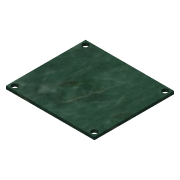
# Autodesk Inventor part: 00_motordriver_pcb
Saved by Autodesk Inventor 2019.4 (Build 234330000, 330)
## iProperties
Created: 2020-06-15
Part Number: 00_motordriver_pcb
Material: Generic
Document SubType Name: Modeling
Designer: diederichbenedict
Density: 1 g/cm^3
Appearance: Green Polished
Author: diederichbenedict
Autodesk Inventor part; units mm, degrees
ref_plane "YZ Plane" through (0, 0, 0) normal (1, 0, 0) x (0, 1, 0)
ref_plane "XZ Plane" through (0, 0, 0) normal (0, 1, 0) x (-1, 0, 0)
ref_plane "XY Plane" through (0, 0, 0) normal (0, 0, 1) x (1, 0, 0)
sketch "Sketch1" plane through (0, 0, 0) normal (0, 1, 0) x (-1, 0, 0)
  line L0 (0, 0) -> (-30, 0)
  line L1 (-30, 0) -> (-30, 27)
  line L2 (-30, 27) -> (0, 27)
  line L3 (0, 27) -> (0, 0)
  dimension "d0" = 30
  dimension "d1" = 27
  constraints: 8 end point, 2 parallel, 1 horizontal, 1 perpendicular
  measures "d0" distance of L1.end L2.end
  measures "d1" distance of L0.end L1.end
extrude "Extrusion1" add sketch "Sketch1" along normal blind 1
sketch "Sketch2" plane through (0, 1, 0) normal (0, 1, 0) x (1, 0, 0)
  line L0 (30, 0) -> (0, 0) projected
  line L1 (0, 0) -> (0, -27) projected
  line L2 (0, -27) -> (30, -27) projected
  line L3 (30, -27) -> (30, 0) projected
  line L4 (1.5, -25.5) -> (1.5, -1.5)
  line L5 (1.5, -1.5) -> (28.5, -1.5)
  line L6 (28.5, -1.5) -> (28.5, -25.5)
  line L7 (28.5, -25.5) -> (1.5, -25.5)
  circle A0 centre (1.5, -25.5) radius 1
  circle A1 centre (28.5, -25.5) radius 1
  circle A2 centre (1.5, -1.5) radius 1
  circle A3 centre (28.5, -1.5) radius 1
  dimension "d4" = 1.5
  dimension "d5" = 2
  dimension "d6" = 2
  dimension "d7" = 2
  dimension "d8" = 2
  constraints: 8 end point, 4 centre point, 4 coincident, 3 other
  measures "d4" distance between parallel lines of L1 L4
  measures "d5" diameter of A0
  measures "d6" diameter of A1
  measures "d7" diameter of A2
  measures "d8" diameter of A3
extrude "Extrusion2" cut sketch "Sketch2" against normal through all contours L7 A0 L4 | L4 A0 L7 | A2 L5 L4 | L4 L5 A2 | A1 L6 L7 | L7 L6 A1 | A3 L6 L5 | L5 L6 A3
body "Solid1"
